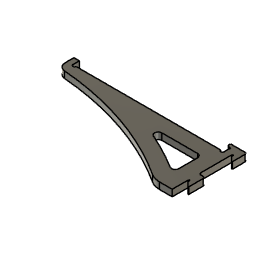
MK2_EU_french_cleat (Autodesk Fusion 360 design; units mm, degrees)
Autodesk Fusion 360 part; units mm, degrees
sketch "Sketch1" plane through (0, 0, 0) normal (0, 0, 1) x (1, 0, 0)
  line L0 (-207.5, 0) -> (207.5, 0) construction
  line L1 (207.5, 0) -> (207.5, 18) construction
  line L2 (207.5, 18) -> (203.5, 18)
  line L3 (203.5, 18) -> (197.5, 22)
  line L4 (197.5, 22) -> (197.5, 28)
  line L5 (197.5, 28) -> (242.5, 28)
  line L6 (242.5, 28) -> (242.5, -14)
  line L7 (242.5, -14) -> (225.5, 3) construction
  line L8 (225.5, 3) -> (225.5, -87)
  line L9 (225.5, -87) -> (242.5, -87)
  line L10 (242.5, -87) -> (242.5, -134)
  line L11 (242.5, -134) -> (225.5, -117) construction
  line L12 (225.5, -117) -> (225.5, -160)
  line L13 (225.5, -160) -> (175.5, -160)
  line L14 (-207.5, 0) -> (-207.5, 18)
  line L15 (-207.5, 18) -> (-222.5, 18)
  line L16 (-222.5, 18) -> (-222.5, -25)
  arc A0 (175.5, -160) -> (-222.5, -25) centre (-271.4526, -823.5009) ccw
  line L17 (242.5, -14) -> (243.5, -15) construction
  line L18 (243.5, -15) -> (243.5, -62) construction
  line L19 (243.5, -62) -> (225.5, -62) construction
  line L20 (242.5, -134) -> (243.5, -135) construction
  line L21 (243.5, -135) -> (243.5, -182) construction
  line L22 (243.5, -182) -> (225.5, -182) construction
  line L23 (225.5, -182) -> (225.5, -160) construction
  line L24 (185.5, -40) -> (185.5, -120)
  line L25 (185.5, -40) -> (25.5, -40)
  arc A1 (185.5, -120) -> (25.5, -40) centre (-250.0278, -791.0556) ccw
  line L26 (225.5, 3) -> (225.5, 4)
  arc A2 (229, 4) -> (225.5, 4) centre (227.25, 4) ccw
  line L27 (229, 4) -> (229, -0.5)
  line L28 (229, -0.5) -> (242.5, -14)
  line L29 (225.5, -117) -> (225.5, -116)
  arc A3 (229, -116) -> (225.5, -116) centre (227.25, -116) ccw
  line L30 (229, -116) -> (229, -120.5)
  line L31 (229, -120.5) -> (242.5, -134)
  arc A4 (207.5, 14.5) -> (207.5, 18) centre (207.5, 16.25) ccw
  line L32 (207.5, 14.5) -> (207.5, 0)
  arc A5 (198.5, 0) -> (207.5, 0) centre (203, 0) ccw
  arc A6 (-207.5, 0) -> (-198.5, 0) centre (-203, 0) ccw
  line L33 (198.5, 0) -> (-198.5, 0)
  dimension "d1" = 415
  dimension "d2" = 15
  dimension "d3" = 10
  dimension "d4" = 4
  dimension "d5" = 4
  dimension "d6" = 45
  dimension "d7" = 25
  dimension "d8" = 17
  dimension "d9" = 25
  dimension "d10" = 18
  dimension "d11" = 45
  dimension "d12" = 45
  dimension "d13" = 120
  dimension "d14" = 65
  dimension "d15" = 65
  dimension "d16" = 163
  dimension "d17" = 50
  dimension "d18" = 25
  dimension "d19" = 800
  dimension "d20" = 18
  dimension "d21" = 207.5
  dimension "d22" = 40
  dimension "d23" = 40
  dimension "d24" = 160
  dimension "d25" = 80
  dimension "d27" = 3.5
  dimension "d28" = 3.5
  dimension "d29" = 1
  dimension "d30" = 10
  dimension "d31" = 3.5
  dimension "d32" = 9
  constraint horizontal L0
  constraint perpendicular L0 L1
  constraint perpendicular L1 L2
  constraint perpendicular L2 L4
  constraint perpendicular L4 L5
  constraint perpendicular L5 L6
  constraint perpendicular L5 L8
  constraint perpendicular L8 L9
  constraint perpendicular L9 L10
  constraint perpendicular L9 L12
  constraint perpendicular L12 L13
  constraint perpendicular L0 L14
  constraint perpendicular L14 L15
  constraint perpendicular L15 L16
  constraint parallel L7 L17
  constraint parallel L6 L18
  constraint coincident L8 L19.end
  constraint perpendicular L8 L19
  constraint collinear L6 L10
  constraint collinear L8 L12
  constraint parallel L11 L20
  constraint parallel L10 L21
  constraint perpendicular L21 L22
  constraint collinear L8 L23
  constraint collinear L18 L21
  constraint coincident origin L0
  constraint collinear L2 L15
  constraint parallel L18 L24
  constraint perpendicular L24 L25
  constraint equal A0 A1
  constraint parallel L8 L26
  constraint tangent L26 A2
  constraint coincident L7 L27.end
  constraint tangent A2 L27
  constraint parallel L26 L27
  constraint parallel L12 L29
  constraint tangent L29 A3
  constraint coincident L11 L30.end
  constraint tangent A3 L30
  constraint parallel L29 L30
  constraint equal L26 L29
  constraint coincident L1 A4.start
  constraint tangent L2 A4
  constraint coincident L0 A5.start
  constraint tangent L1 A5
  constraint coincident L0 A6.end
  constraint tangent L14 A6
  constraint equal A5 A6
  measures "d1" distance of L1 L14
  measures "d2" distance of L14.end L15.end
  measures "d3" distance of L2 L5
  measures "d4" distance of L1 L2.end
  measures "d5" distance of L2 L3.end
  measures "d6" distance of L4 L6
  measures "d7" distance of L5 L7.end
  measures "d8" distance of L6 L8
  measures "d9" distance of L9 L19
  measures "d10" distance of L8 L18
  measures "d11" angle of L7 L8
  measures "d12" angle of L11 L12
  measures "d13" distance of L19 L22
  measures "d14" distance of L7.end L19
  measures "d15" distance of L11.end L22
  measures "d16" distance of L7.end L13
  measures "d17" distance of L12.end L13.end
  measures "d18" distance of L0 L16.end
  measures "d19" radius of A0
  measures "d20" distance of L0 L2
  measures "d21" distance of origin L14
  measures "d22" distance of L0 L25
  measures "d23" distance of L8 L24
  measures "d24" distance of L24.start L25.end
  measures "d25" distance of L24.start L24.end
  measures "d27" diameter of A2
  measures "d28" diameter of A3
  measures "d29" distance of L7.end L26.end
  measures "d30" distance of L1 L4
  measures "d31" diameter of A4
  measures "d32" diameter of A5
extrude "Extrude1" add sketch "Sketch1" along normal blind 18
fillet "Fillet1" radius 1 6 edges at (242.5, -14, 9) (242.5, -134, 9) (229, -120.5, 9) (229, -0.5, 9) (197.5, 28, 9) (197.5, 22, 9)
fillet "Fillet1" radius 20 1 edges at (-222.5, -25, 9)
fillet "Fillet1" radius 10 3 edges at (185.5, -40, 9) (185.5, -120, 9) (25.5, -40, 9)
fillet "Fillet1" radius 50 1 edges at (175.5, -160, 9)
fillet "Fillet1" radius 5 3 edges at (242.5, 28, 9) (242.5, -87, 9) (225.5, -87, 9)
fillet "Fillet1" radius 5 1 edges at (203.5, 18, 9)
equation "d12 = d11"
equation "d13 = 55 mm + 65 mm"
equation "d15 = d14"
equation "d21 = d1 / 2"
equation "d28 = d27"
equation "d31 = d27"
